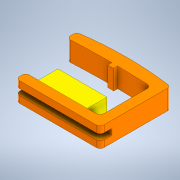
# Autodesk Inventor part: pogo-holder-base
Saved by Autodesk Inventor 2021 (Build 250183000, 183)
## iProperties
Created: 2021-09-24
Part Number: pogo-holder-base
Material: Generic
Document SubType Name: Modeling
Designer: caleb
Density: 1 g/cm^3
Appearance: Default
Author: caleb
Autodesk Inventor part; units mm, degrees
ref_plane "YZ Plane" through (0, 0, 0) normal (1, 0, 0) x (0, 1, 0)
ref_plane "XZ Plane" through (0, 0, 0) normal (0, 1, 0) x (-1, 0, 0)
ref_plane "XY Plane" through (0, 0, 0) normal (0, 0, 1) x (1, 0, 0)
sketch "Sketch1" plane through (0, 0, 0) normal (0, 0, 1) x (1, 0, 0)
  line L0 (-5.09, 0) -> (5.09, 0) construction
  line L1 (-7.74, 0) -> (-5.09, 0) construction
  line L2 (5.09, 0) -> (7.74, 0) construction
  line L3 (-12.5, -5) -> (12.5, -5)
  line L4 (12.5, -5) -> (12.5, 5)
  line L5 (12.5, 5) -> (-12.5, 5)
  line L6 (-12.5, 5) -> (-12.5, -5)
  point P0 (0, 0)
  point P1 (0, 0)
  point P2 (-12.5, 0)
  point P3 (0, 5)
  dimension "d0" = 2.65
  dimension "d1" = 12.83
  dimension "d2" = 25
  dimension "d3" = 10
  constraints: 14 end point, 4 horizontal, 3 coincident, 3 midpoint, 2 parallel, 1 collinear, 1 horizontal alignment, 1 perpendicular, 1 point on line, 1 vertical alignment
  measures "d0" distance of L1.start L1.end
  measures "d1" distance of L0.end L1.start
  measures "d2" distance of L3.start L3.end
  measures "d3" distance of L3.end L4.end
extrude "Extrusion1" add sketch "Sketch1" along normal blind 10
hole "Hole1" at (-5.09, 0, 0) at (5.09, 0, 0) at (7.74, 0, 0) at (-7.74, 0, 0) direction (0, 0, 1) diameter 1.7 end through all
sketch "Sketch2" plane through (-12.5, 5, 0) normal (0, 1, 0) x (1, 0, 0)
  line L0 (25, 0) -> (0, 0) construction
  line L1 (0, 0) -> (0, -10) construction
  line L2 (25, -10) -> (0, -10) construction
  line L3 (25, 0) -> (25, -10) construction
  line L4 (-6.5, -10) -> (-6.5, -15)
  line L5 (-6.5, -15) -> (36.5, -15)
  line L6 (36.5, -15) -> (36.5, 20.9046)
  arc A0 (36.5, 20.9046) -> (-11.5, 20.9046) centre (12.5, -139.5491) ccw
  arc A1 (31.5, 15.9046) -> (-11.5, 15.9046) centre (10, -366.7641) ccw
  line L7 (-6.5, -10) -> (31.5, -10)
  line L8 (25, -10) -> (0, -10) projected
  line L9 (12.5, 0) -> (12.5, 16.5) construction
  line L10 (25, 0) -> (0, 0) projected
  line L11 (31.5, 15.9046) -> (31.5, -10)
  line L12 (-11.5, 20.9046) -> (-11.5, 15.9046)
  point P0 (12.5, -10)
  point P1 (12.5, -10)
  dimension "d13" = 38
  dimension "d15" = 5
  dimension "d16" = 5
  dimension "d18" = 16.5
  dimension "d19" = 5
  dimension "d20" = 383.2723
  dimension "d21" = 162.2388
  constraints: 14 end point, 5 point on circle, 3 midpoint, 3 perpendicular, 3 vertical, 2 centre point, 2 horizontal alignment, 1 horizontal, 1 vertical alignment
  measures "d13" distance of L4.start L7.end
  measures "d15" distance between parallel lines of L5 L7
  measures "d16" distance of L12.start L12.end
  measures "d18" distance of L9.start L9.end
  measures "d19" distance between parallel lines of L6 L11
  measures "d20" radius of A1
  measures "d21" radius of A0
extrude "Extrusion2" add sketch "Sketch2" against normal up to surface (10 mm away) separate body
sketch "Sketch3" plane through (-12.5, 5, 0) normal (0, 1, 0) x (1, 0, 0)
  arc A0 (31.5, 15.9046) -> (-11.5, 15.9046) centre (10, -366.7641) ccw projected
  line L0 (11, 14.4873) -> (14, 14.4873)
  line L1 (14, 14.4873) -> (14, 16.4873)
  line L2 (11, 14.4873) -> (11, 16.5068)
  line L3 (25, 0) -> (0, 0) projected
  point P0 (12.5, 0)
  point P1 (12.5, 14.4873)
  point P2 (12.5, 0)
  dimension "d24" = 2
  dimension "d25" = 3
  constraints: 6 end point, 2 midpoint, 2 point on circle, 1 horizontal, 1 parallel, 1 perpendicular, 1 vertical alignment
  measures "d24" distance of L0.end L1.end
  measures "d25" distance of L0.start L0.end
extrude "Extrusion3" add sketch "Sketch3" against normal up to surface (10 mm away) bodies 2
fillet "Fillet1" radius 2 8 edges at (19, 0, -15.9046) (19, 0, 10) (24, 0, 15) (24, 0, -20.9046) (-24, 0, -15.9046) (-24, 0, -20.9046) (-19, 0, 10) (-19, 0, 15)
sketch "Sketch4" plane through (-17, 5, 15) normal (0, 0, 1) x (1, 0, 0)
  line L0 (0, -10) -> (0, 0) construction
  line L1 (0, -10) -> (39, -10) construction
  line L2 (39, 0) -> (39, -10) construction
  line L3 (0, 0) -> (39, 0) construction
  line L4 (-7, -3.5) -> (41, -3.5)
  line L5 (41, -3.5) -> (41, -6.5)
  line L6 (41, -6.5) -> (-7, -6.5)
  line L7 (-7, -6.5) -> (-7, -3.5)
  line L8 (41, -10) -> (41, 0) projected
  line L9 (-7, 0) -> (-7, -10) projected
  point P0 (17, -5)
  point P1 (41, -5)
  point P2 (39, -5)
  dimension "d29" = 3
  constraints: 8 end point, 2 midpoint, 2 parallel, 2 point on line, 1 horizontal, 1 horizontal alignment, 1 perpendicular
  measures "d29" distance of L4.end L5.end
extrude "Extrusion4" cut sketch "Sketch4" against normal blind 5.75 bodies 2
body "Solid1"
body "Solid2"
